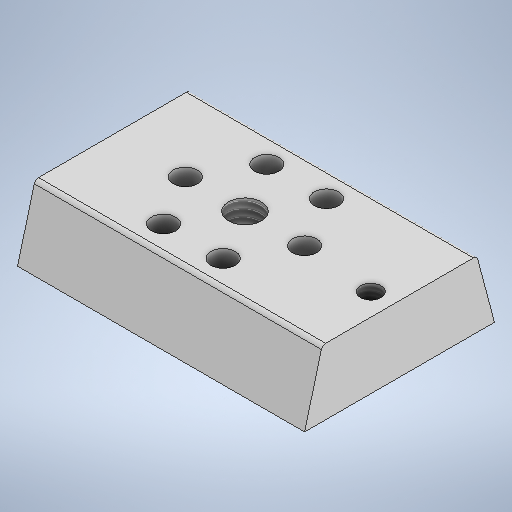
# Autodesk Inventor part: Wedge-Dove tail
Saved by Autodesk Inventor 2025 (Build 290162000, 162)
## iProperties
Created: 2025-08-11
Part Number: Wedge-Dove tail
Material: Generic
Document SubType Name: Modeling
Designer: yshis
Density: 1 g/cm^3
Appearance: Default
Author: yshis
Autodesk Inventor part; units mm, degrees
ref_plane "YZ Plane" through (0, 0, 0) normal (1, 0, 0) x (0, 1, 0)
ref_plane "XZ Plane" through (0, 0, 0) normal (0, 1, 0) x (-1, 0, 0)
ref_plane "XY Plane" through (0, 0, 0) normal (0, 0, 1) x (1, 0, 0)
sketch "Sketch1" plane through (0, 0, 0) normal (0, 1, 0) x (-1, 0, 0)
  line L0 (0, 0) -> (65, 0)
  line L1 (65, 0) -> (65, -43)
  line L2 (65, -43) -> (0, -43)
  line L3 (0, -43) -> (0, 0)
  dimension "d0" = 65
  dimension "d1" = 43
  constraints: 8 end point, 2 parallel, 1 horizontal, 1 perpendicular
  measures "d0" distance of L1.end L2.end
  measures "d1" distance of L0.end L1.end
extrude "Extrusion1" add sketch "Sketch1" along normal blind 15
sketch "Sketch2" plane through (0, 0, 0) normal (0, -1, 0) x (1, 0, 0)
  line L0 (-55, -36.5) -> (-15, -36.5)
  line L1 (-10, -31.5) -> (-10, -11.5)
  line L2 (-15, -6.5) -> (-55, -6.5)
  line L3 (-60, -11.5) -> (-60, -31.5)
  line L4 (-65, 0) -> (0, 0) projected
  line L5 (0, -43) -> (-65, -43) projected
  line L6 (0, 0) -> (0, -43) projected
  line L7 (-65, -43) -> (-65, 0) projected
  arc A0 (-10, -11.5) -> (-15, -6.5) centre (-15, -11.5) ccw
  arc A1 (-55, -6.5) -> (-60, -11.5) centre (-55, -11.5) ccw
  arc A2 (-60, -31.5) -> (-55, -36.5) centre (-55, -31.5) ccw
  arc A3 (-15, -36.5) -> (-10, -31.5) centre (-15, -31.5) ccw
  dimension "d4" = 6.5
  dimension "d5" = 6.5
  dimension "d6" = 10
  dimension "d7" = 5
  dimension "d8" = 5
  constraints: 8 end point, 8 point on circle, 8 tangent, 4 centre point, 3 equal radius, 2 parallel, 1 horizontal, 1 perpendicular
  measures "d4" distance between parallel lines of L4 L2
  measures "d5" distance between parallel lines of L5 L0
  measures "d6" distance between parallel lines of L6 L1
  measures "d7" distance between parallel lines of L7 L3
  measures "d8" radius of A0
extrude "Extrusion2" cut sketch "Sketch2" against normal blind 7 contours A2 L3 A1 L2 A0 L1 A3 L0
sketch "Sketch3" plane through (0, 7, 0) normal (0, -1, 0) x (1, 0, 0)
  circle A0 centre (-35, -21.5) radius 3.75
  line L0 (-10, -11.5) -> (-10, -31.5) projected
  line L1 (-15, -36.5) -> (-55, -36.5) projected
  point P0 (0, 0)
  dimension "d11" = 7.5
  dimension "d12" = 25
  dimension "d13" = 15
  constraints: 1 centre point
  measures "d11" diameter of A0
  measures "d12" distance from line of A0.centre L0
  measures "d13" distance from line of A0.centre L1
extrude "Extrusion3" cut sketch "Sketch3" against normal blind 8
thread "Thread1" size "3/8-16 UNC" class "2B" standard "ANSI Unified Screw Threads" full length
sketch "Sketch4" plane through (0, 0, 0) normal (0, -1, 0) x (1, 0, 0)
  circle A0 centre (-5, -20) radius 2.35
  line L0 (-65, 0) -> (0, 0) projected
  line L1 (0, 0) -> (0, -43) projected
  dimension "d18" = 4.7
  dimension "d19" = 20
  dimension "d20" = 5
  constraints: 1 centre point
  measures "d18" diameter of A0
  measures "d19" distance from line of A0.centre L0
  measures "d20" distance from line of A0.centre L1
extrude "Extrusion4" cut sketch "Sketch4" against normal blind 15
thread "Thread2" size "12-24 UNC" class "2B" standard "ANSI Unified Screw Threads" full length
chamfer "Chamfer1" distance 4 distance2 15 2 edges at (-32.5, 15, -43) (-32.5, 15, 0) measured on face at (-33.1827, 15, -37.0742)
fillet "Fillet1" radius 1 2 edges at (-32.5, 15, -39.0005) (-32.5, 15, -3.9995)
sketch "Sketch5" plane through (0, 15, 0) normal (0, 1, 0) x (1, 0, 0)
  circle A0 centre (-21.5, 21.5) radius 2.75
  circle A1 centre (-35, 21.5) radius 3.75 projected
  circle A2 centre (-28.25, 33.1913) radius 2.75
  circle A3 centre (-41.75, 33.1913) radius 2.75
  circle A4 centre (-48.5, 21.5) radius 2.75
  circle A5 centre (-41.75, 9.8087) radius 2.75
  circle A6 centre (-28.25, 9.8087) radius 2.75
  point P0 (0, 0)
  dimension "d29" = 5.5
  dimension "d30" = 13.5
  dimension "d33" = 360
  constraints: 6 centre point, 13 other
  measures "d29" diameter of A0
  measures "d30" distance of A0.centre A1.centre
extrude "Extrusion5" cut sketch "Sketch5" against normal blind 15 contours A0 | A2 | A3 | A4 | A5 | A6
body "Solid1"
